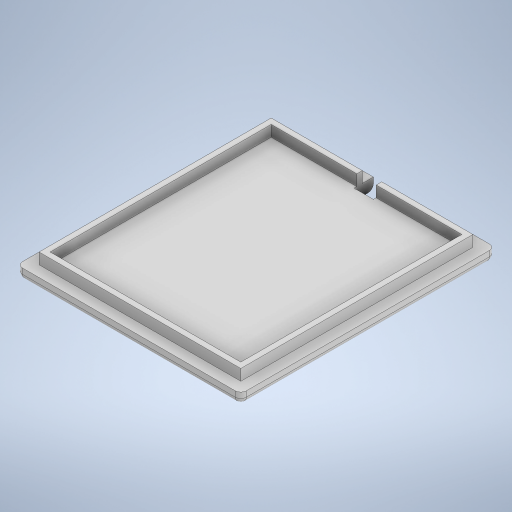
# Autodesk Inventor part: Battery Box Lid
Saved by Autodesk Inventor 2024 (Build 280153000, 153)
## iProperties
Created: 2023-07-26
Part Number: Battery Box Lid
Material: Generic
Document SubType Name: Modeling
Designer: techn
Density: 1 g/cm^3
Appearance: Default
Author: techn
## iProperties of the stored document Battery Box Lid_3DPrint.ipt
Created: 2023-07-26
Part Number: Battery Box Lid_3DPrint
Material: Generic
Document SubType Name: Modeling
Designer: techn
Density: 1 g/cm^3
Appearance: Default
Author: techn
Autodesk Inventor part; units mm, degrees
ref_plane "YZ Plane" through (0, 0, 0) normal (1, 0, 0) x (0, 1, 0)
ref_plane "XZ Plane" through (0, 0, 0) normal (0, 1, 0) x (-1, 0, 0)
ref_plane "XY Plane" through (0, 0, 0) normal (0, 0, 1) x (1, 0, 0)
sketch "Sketch1" plane through (0, 0, 0) normal (0, 1, 0) x (-1, 0, 0)
  line L0 (6.21, 11.0673) -> (-74.79, 11.0673)
  line L1 (-74.79, 11.0673) -> (-74.79, -80.9327)
  line L2 (-74.79, -80.9327) -> (6.21, -80.9327)
  line L3 (6.21, -80.9327) -> (6.21, 11.0673)
  point P0 (0, 0)
  dimension "d0" = 81
  dimension "d1" = 92
  constraints: 8 end point, 2 parallel, 1 horizontal, 1 perpendicular
  measures "d0" distance of L2.end L1.end
  measures "d1" distance of L1.end L0.end
extrude "Extrusion1" add sketch "Sketch1" along normal blind 4
sketch "Sketch2" plane through (0, 4, 0) normal (0, 1, 0) x (1, 0, 0)
  line L0 (-6.21, -11.0673) -> (74.79, -11.0673) projected
  line L1 (-3.1343, -11.0673) -> (0.8657, -11.0673) construction
  line L2 (-6.21, 80.9327) -> (-6.21, -11.0673) projected
  line L3 (-2.21, -7.0673) -> (70.79, -7.0673)
  line L4 (70.79, -7.0673) -> (70.79, 76.9327)
  line L5 (70.79, 76.9327) -> (-2.21, 76.9327)
  line L6 (-2.21, 76.9327) -> (-2.21, -7.0673)
  line L7 (74.79, -11.0673) -> (74.79, 80.9327) projected
  line L8 (-6.21, -11.0673) -> (74.79, -11.0673)
  line L9 (74.79, -11.0673) -> (74.79, 80.9327)
  line L10 (74.79, 80.9327) -> (-6.21, 80.9327)
  line L11 (-6.21, 80.9327) -> (-6.21, -11.0673)
  line L12 (-6.21, 80.9327) -> (-6.21, -11.0673) projected
  line L13 (2.4089, -7.0673) -> (4.4089, -7.0673) construction
  line L14 (-2.21, -5.0673) -> (-0.21, -5.0673) construction
  line L15 (-0.21, -5.0673) -> (68.79, -5.0673)
  line L16 (68.79, -5.0673) -> (68.79, 74.9327)
  line L17 (68.79, 74.9327) -> (-0.21, 74.9327)
  line L18 (-0.21, 74.9327) -> (-0.21, -5.0673)
  point P0 (0, 0)
  dimension "d8" = 73
  dimension "d9" = 84
  dimension "d14" = 69
  dimension "d15" = 80
  constraints: 30 end point, 6 horizontal, 6 parallel, 3 perpendicular, 3 point on line
  measures "d8" distance of L5.end L4.end
  measures "d9" distance of L4.end L3.end
  measures "d14" distance of L17.end L16.end
  measures "d15" distance of L16.end L15.end
extrude "Extrusion2" add sketch "Sketch2" along normal blind 4 contours L6 L5 L4 L3
sketch "Sketch3" plane through (0, 4, 0) normal (0, 1, 0) x (1, 0, 0)
  line L0 (-6.21, 80.9327) -> (-6.21, -11.0673) projected
  line L1 (-6.21, 78.6108) -> (34.29, 78.6108)
  line L2 (74.79, -11.0673) -> (74.79, 80.9327) projected
  line L3 (34.29, 78.6108) -> (34.29, 76.9327)
  line L4 (70.79, 76.9327) -> (-2.21, 76.9327) projected
  line L5 (34.29, 76.9327) -> (30.79, 76.9327)
  line L6 (30.79, 76.9327) -> (34.29, 76.9327)
  line L7 (34.29, 76.9327) -> (37.79, 76.9327)
  line L8 (37.79, 76.9327) -> (37.79, 73.9327)
  line L9 (37.79, 73.9327) -> (30.79, 73.9327)
  line L10 (30.79, 73.9327) -> (30.79, 76.9327)
  point P0 (0, 0)
  dimension "d18" = 40.5
  dimension "d19" = 3.5
  dimension "d20" = 3.5
  dimension "d21" = 3.5
  dimension "d22" = 3
  dimension "d23" = 7
  constraints: 16 end point, 3 perpendicular, 3 point on line, 1 collinear, 1 midpoint
  measures "d18" distance of L1.start L1.end
  measures "d19" distance of L3.end L5.end
  measures "d20" distance of L5.end L3.end
  measures "d21" distance of L3.end L7.end
  measures "d22" distance of L7.end L8.end
  measures "d23" distance of L8.end L9.end
extrude "Extrusion3" cut sketch "Sketch3" against normal blind 4
sketch "Sketch4" plane through (0, 4, 0) normal (0, -1, 0) x (1, 0, 0)
  line L0 (30.79, -76.9327) -> (37.79, -76.9327) projected
  line L1 (30.79, -73.9327) -> (30.79, -74.9327) projected
  line L2 (37.79, -76.9327) -> (30.79, -76.9327)
  line L3 (30.79, -76.9327) -> (30.79, -74.9327)
  line L4 (30.79, -74.9327) -> (37.79, -74.9327)
  line L5 (37.79, -74.9327) -> (37.79, -76.9327)
  point P0 (0, 0)
  constraints: 8 end point, 2 parallel, 1 horizontal, 1 perpendicular
extrude "Extrusion4" cut sketch "Sketch4" against normal blind 10
sketch "Sketch5" plane through (30.79, 4, -76.9327) normal (0, 0, 1) x (1, 0, 0)
  line L0 (7, -4) -> (0, -4) projected
  line L1 (0, 0) -> (0, -4) projected
  line L2 (7, -4) -> (0, -4)
  line L3 (0, -4) -> (0, 0)
  line L4 (0, 0) -> (7, 0)
  line L5 (7, 0) -> (7, -4)
  point P0 (-30.79, -4)
  constraints: 8 end point, 2 parallel, 1 horizontal, 1 perpendicular
extrude "Extrusion5" cut sketch "Sketch5" against normal blind 10
fillet "Fillet1" radius 2 9 edges at (74.79, 2, 11.0673) (74.79, 0, -34.9327) (34.29, 0, 11.0673) (-6.21, 2, 11.0673) (-6.21, 0, -34.9327) (-6.21, 2, -80.9327) (12.29, 0, -80.9327) (56.29, 0, -80.9327) (74.79, 2, -80.9327)
body "Solid1"
